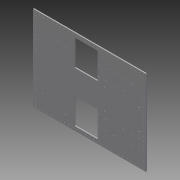
# Autodesk Inventor part: uderbodyweight
Saved by Autodesk Inventor 2014 SP1 (Build 180222100, 222)
## iProperties
Created: 2014-01-07
Part Number: uderbodyweight
Material: Steel
Document SubType Name: Modeling
Designer: Arpan
Density: 7.85 g/cm^3
Appearance: Steel
Mass: 15333 g
Surface Area: 6502.64 cm^2
Volume: 1953.25 cm^3
Author: Arpan
Autodesk Inventor part; units mm, degrees
ref_plane "YZ Plane" through (0, 0, 0) normal (1, 0, 0) x (0, 1, 0)
ref_plane "XZ Plane" through (0, 0, 0) normal (0, 1, 0) x (-1, 0, 0)
ref_plane "XY Plane" through (0, 0, 0) normal (0, 0, 1) x (1, 0, 0)
sketch "Sketch1" plane through (0, 0, 0) normal (0, 0, 1) x (1, 0, 0)
  circle A0 centre (435.0722, 321.6304) radius 3.2639
  circle A1 centre (198.3647, 418.811) radius 2.5119
  circle A2 centre (440.3741, 420.236) radius 2.1989
  circle A3 centre (542.5208, 420.236) radius 2.1989
  circle A4 centre (644.6428, 420.236) radius 2.1989
  circle A5 centre (491.4414, 357.8965) radius 2.1989
  circle A6 centre (593.5881, 357.8965) radius 2.1989
  circle A7 centre (398.5657, 358.1076) radius 2.1723
  circle A8 centre (500.7124, 358.1076) radius 2.1723
  circle A9 centre (602.8344, 358.1076) radius 2.1723
  circle A10 centre (449.633, 420.0249) radius 2.1723
  circle A11 centre (551.7797, 420.0249) radius 2.1723
  circle A12 centre (644.6222, 194.6304) radius 3.2639
  circle A13 centre (57.15, 98.044) radius 2.4116
  circle A14 centre (197.0948, 59.563) radius 2.4116
  circle A15 centre (542.5208, 158.3585) radius 2.1989
  circle A16 centre (491.4414, 158.3585) radius 2.1989
  circle A17 centre (440.3741, 96.019) radius 2.1989
  circle A18 centre (542.5208, 96.019) radius 2.1989
  circle A19 centre (644.6428, 96.019) radius 2.1989
  circle A20 centre (449.633, 96.2301) radius 2.1723
  circle A21 centre (500.7124, 96.2301) radius 2.1723
  circle A22 centre (398.5657, 158.1474) radius 2.1723
  circle A23 centre (500.7124, 158.1474) radius 2.1723
  circle A24 centre (602.8344, 158.1474) radius 2.1723
  circle A25 centre (551.7797, 158.1474) radius 2.1723
  circle A26 centre (449.633, 158.1474) radius 2.1723
  circle A27 centre (398.5657, 96.2301) radius 2.1723
  circle A28 centre (551.7797, 96.2301) radius 2.1723
  circle A29 centre (602.8344, 96.2301) radius 2.1723
  circle A30 centre (593.5881, 96.019) radius 2.1989
  circle A31 centre (491.4414, 96.019) radius 2.1989
  circle A32 centre (593.5881, 158.3585) radius 2.1989
  circle A33 centre (440.3741, 158.3585) radius 2.1989
  circle A34 centre (644.6428, 158.3585) radius 2.1989
  circle A35 centre (197.0948, 95.631) radius 2.4116
  circle A36 centre (57.15, 57.15) radius 2.4116
  circle A37 centre (435.0722, 194.6304) radius 3.2639
  circle A38 centre (602.8344, 420.0249) radius 2.1723
  circle A39 centre (500.7124, 420.0249) radius 2.1723
  circle A40 centre (398.5657, 420.0249) radius 2.1723
  circle A41 centre (551.7797, 358.1076) radius 2.1723
  circle A42 centre (449.633, 358.1076) radius 2.1723
  circle A43 centre (644.6428, 357.8965) radius 2.1989
  circle A44 centre (542.5208, 357.8965) radius 2.1989
  circle A45 centre (440.3741, 357.8965) radius 2.1989
  circle A46 centre (593.5881, 420.236) radius 2.1989
  circle A47 centre (491.4414, 420.236) radius 2.1989
  circle A48 centre (151.1207, 418.811) radius 2.5119
  circle A49 centre (644.6222, 321.6304) radius 3.2639
  circle A50 centre (12.7, 486.7275) radius 2.0701
  circle A51 centre (12.7, 461.3275) radius 2.0701
  circle A52 centre (12.7, 435.9275) radius 2.0701
  circle A53 centre (12.7, 410.5275) radius 2.0701
  circle A54 centre (12.7, 385.1275) radius 2.0701
  circle A55 centre (12.7, 359.7275) radius 2.0701
  circle A56 centre (12.7, 334.3275) radius 2.0701
  circle A57 centre (12.7, 308.9275) radius 2.0701
  circle A58 centre (12.7, 283.5275) radius 2.0701
  circle A59 centre (12.7, 258.1275) radius 2.0701
  circle A60 centre (12.7, 232.7275) radius 2.0701
  circle A61 centre (12.7, 207.3275) radius 2.0701
  circle A62 centre (12.7, 181.9275) radius 2.0701
  circle A63 centre (12.7, 156.5275) radius 2.0701
  circle A64 centre (12.7, 131.1275) radius 2.0701
  circle A65 centre (12.7, 105.7275) radius 2.0701
  circle A66 centre (12.7, 80.3275) radius 2.0701
  circle A67 centre (12.7, 54.9275) radius 2.0701
  circle A68 centre (12.7, 29.5275) radius 2.0701
  circle A69 centre (673.1, 486.7275) radius 2.0701
  circle A70 centre (673.1, 461.3275) radius 2.0701
  circle A71 centre (673.1, 435.9275) radius 2.0701
  circle A72 centre (673.1, 410.5275) radius 2.0701
  circle A73 centre (673.1, 385.1275) radius 2.0701
  circle A74 centre (673.1, 359.7275) radius 2.0701
  circle A75 centre (673.1, 334.3275) radius 2.0701
  circle A76 centre (673.1, 308.9275) radius 2.0701
  circle A77 centre (673.1, 283.5275) radius 2.0701
  circle A78 centre (673.1, 258.1275) radius 2.0701
  circle A79 centre (673.1, 232.7275) radius 2.0701
  circle A80 centre (673.1, 207.3275) radius 2.0701
  circle A81 centre (673.1, 181.9275) radius 2.0701
  circle A82 centre (673.1, 156.5275) radius 2.0701
  circle A83 centre (673.1, 131.1275) radius 2.0701
  circle A84 centre (673.1, 105.7275) radius 2.0701
  circle A85 centre (673.1, 80.3275) radius 2.0701
  circle A86 centre (673.1, 54.9275) radius 2.0701
  circle A87 centre (673.1, 29.5275) radius 2.0701
  line L0 (252.73, 332.105) -> (252.73, 490.855)
  line L1 (252.73, 490.855) -> (392.43, 490.855)
  line L2 (392.43, 490.855) -> (392.43, 332.105)
  line L3 (392.43, 332.105) -> (252.73, 332.105)
  line L4 (392.43, 25.4) -> (252.73, 25.4)
  line L5 (252.73, 25.4) -> (252.73, 184.15)
  line L6 (252.73, 184.15) -> (392.43, 184.15)
  line L7 (392.43, 184.15) -> (392.43, 25.4)
  circle A88 centre (12.7, 503.555) radius 2.0828
  circle A89 centre (12.7, 12.7) radius 2.0828
  circle A90 centre (38.1, 503.555) radius 2.0828
  circle A91 centre (38.1, 12.7) radius 2.0828
  circle A92 centre (63.5, 503.555) radius 2.0828
  circle A93 centre (63.5, 12.7) radius 2.0828
  circle A94 centre (88.9, 503.555) radius 2.0828
  circle A95 centre (88.9, 12.7) radius 2.0828
  circle A96 centre (114.3, 503.555) radius 2.0828
  circle A97 centre (114.3, 12.7) radius 2.0828
  circle A98 centre (139.7, 503.555) radius 2.0828
  circle A99 centre (139.7, 12.7) radius 2.0828
  circle A100 centre (165.1, 503.555) radius 2.0828
  circle A101 centre (165.1, 12.7) radius 2.0828
  circle A102 centre (190.5, 503.555) radius 2.0828
  circle A103 centre (190.5, 12.7) radius 2.0828
  circle A104 centre (215.9, 503.555) radius 2.0828
  circle A105 centre (215.9, 12.7) radius 2.0828
  circle A106 centre (241.3, 503.555) radius 2.0828
  circle A107 centre (241.3, 12.7) radius 2.0828
  circle A108 centre (266.7, 503.555) radius 2.0828
  circle A109 centre (266.7, 12.7) radius 2.0828
  circle A110 centre (292.1, 503.555) radius 2.0828
  circle A111 centre (292.1, 12.7) radius 2.0828
  circle A112 centre (317.5, 503.555) radius 2.0828
  circle A113 centre (317.5, 12.7) radius 2.0828
  circle A114 centre (342.9, 503.555) radius 2.0828
  circle A115 centre (342.9, 12.7) radius 2.0828
  circle A116 centre (368.3, 503.555) radius 2.0828
  circle A117 centre (368.3, 12.7) radius 2.0828
  circle A118 centre (393.7, 503.555) radius 2.0828
  circle A119 centre (393.7, 12.7) radius 2.0828
  circle A120 centre (419.1, 503.555) radius 2.0828
  circle A121 centre (419.1, 12.7) radius 2.0828
  circle A122 centre (444.5, 503.555) radius 2.0828
  circle A123 centre (444.5, 12.7) radius 2.0828
  circle A124 centre (469.9, 503.555) radius 2.0828
  circle A125 centre (469.9, 12.7) radius 2.0828
  circle A126 centre (495.3, 503.555) radius 2.0828
  circle A127 centre (495.3, 12.7) radius 2.0828
  circle A128 centre (520.7, 503.555) radius 2.0828
  circle A129 centre (520.7, 12.7) radius 2.0828
  circle A130 centre (546.1, 503.555) radius 2.0828
  circle A131 centre (546.1, 12.7) radius 2.0828
  circle A132 centre (571.5, 503.555) radius 2.0828
  circle A133 centre (571.5, 12.7) radius 2.0828
  circle A134 centre (596.9, 503.555) radius 2.0828
  circle A135 centre (596.9, 12.7) radius 2.0828
  circle A136 centre (622.3, 503.555) radius 2.0828
  circle A137 centre (622.3, 12.7) radius 2.0828
  circle A138 centre (647.7, 503.555) radius 2.0828
  circle A139 centre (647.7, 12.7) radius 2.0828
  circle A140 centre (673.1, 503.555) radius 2.0828
  circle A141 centre (673.1, 12.7) radius 2.0828
  line L8 (0, 0) -> (685.8, 0)
  line L9 (685.8, 0) -> (685.8, 516.255)
  line L10 (685.8, 516.255) -> (0, 516.255)
  line L11 (0, 516.255) -> (0, 0)
  constraints: 142 centre point, 24 end point
extrude "Extrusion1" add sketch "Sketch1" along normal blind 6.35
body "Solid1"
